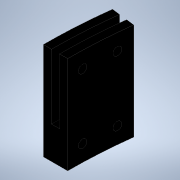
# Autodesk Inventor part: Shield Fastener
Saved by Autodesk Inventor 2020 (Build 240168000, 168)
## iProperties
Created: 2021-01-17
Part Number: Shield Fastener
Material: Generic
Document SubType Name: Modeling
Designer: magda
Density: 1 g/cm^3
Appearance: Default
Author: magda
Autodesk Inventor part; units mm, degrees
ref_plane "YZ Plane" through (0, 0, 0) normal (1, 0, 0) x (0, 1, 0)
ref_plane "XZ Plane" through (0, 0, 0) normal (0, 1, 0) x (-1, 0, 0)
ref_plane "XY Plane" through (0, 0, 0) normal (0, 0, 1) x (1, 0, 0)
sketch "Sketch1" plane through (0, 0, 0) normal (0, 1, 0) x (-1, 0, 0)
  arc A0 (207.988, -25.5377) -> (209.55, 0) centre (0, 0) ccw
  arc A1 (201.6854, -24.7639) -> (203.2, 0) centre (0, 0) ccw
  arc A2 (204.8367, -25.1508) -> (206.375, 0) centre (0, 0) ccw
  arc A3 (198.534, -24.3769) -> (200.025, 0) centre (0, 0) ccw
  line L0 (209.55, 0) -> (200.025, 0)
  line L1 (198.534, -24.3769) -> (207.988, -25.5377)
  dimension "d0" = 419.1
  dimension "d1" = 406.4
  dimension "d2" = 412.75
  dimension "d3" = 400.05
  dimension "d4" = 7
  constraints: 8 point on circle, 4 centre point, 4 coincident, 4 end point, 4 point on line, 1 horizontal
  measures "d0" diameter of A0
  measures "d1" diameter of A1
  measures "d2" diameter of A2
  measures "d3" diameter of A3
  measures "d4" angle of L1 L0
extrude "Extrusion1" add sketch "Sketch1" along normal blind 25.4 contours L1 A2 L0 A0 | L1 A3 L0 A1
ref_plane "Work Plane1" through (0, 0, 0) normal (0, -1, 0) x (1, 0, 0)
sketch "Sketch2" plane through (0, 0, 0) normal (0, -1, 0) x (1, 0, 0)
  line L0 (-203.2, 0) -> (-200.025, 0) projected
  line L1 (-209.55, 0) -> (-206.375, 0) projected
  line L2 (-200.025, 0) -> (-209.55, 0)
  line L3 (-204.8367, -25.1508) -> (-207.988, -25.5377) projected
  arc A0 (-200.025, 0) -> (-198.534, -24.3769) centre (0, 0) ccw projected
  line L4 (-207.988, -25.5377) -> (-198.534, -24.3769)
  arc A1 (-200.025, 0) -> (-198.534, -24.3769) centre (3.1749, 0.1942) ccw
  arc A2 (-209.55, 0) -> (-207.988, -25.5377) centre (0, 0) ccw projected
  arc A3 (-209.55, 0) -> (-207.988, -25.5377) centre (3.1749, 0.1942) ccw
  point P0 (-207.988, -25.5377)
  point P1 (-209.55, 0)
  constraints: 4 end point, 4 point on circle, 2 centre point, 1 collinear
extrude "Extrusion2" add sketch "Sketch2" along normal blind 12.7 contours L0 A0 L4 L3 A3 L1 L2 | A3 A2
ref_plane "Work Plane2" through (-209.55, 0, 0) normal (-0.9981348, 0, -0.0610485) x (0, 1, 0)
sketch "Sketch3" plane through (-209.55, 0, 0) normal (-0.9981348, 0, -0.0610485) x (0, 1, 0)
  circle A0 centre (19.05, 6.35) radius 1.5875
  circle A1 centre (19.05, 19.2354) radius 1.5875
  line L0 (25.4, 0) -> (-12.7, 0) projected
  line L1 (-12.7, 25.5854) -> (25.4, 25.5854) projected
  line L2 (25.4, 0) -> (25.4, 25.5854) projected
  circle A2 centre (-6.35, 19.2354) radius 1.5875
  circle A3 centre (-6.35, 6.35) radius 1.5875
  line L3 (-12.7, 25.5854) -> (-12.7, 0) projected
  point P0 (0, 12.7927)
  dimension "d10" = 3.175
  dimension "d11" = 3.175
  dimension "d12" = 6.35
  dimension "d13" = 6.35
  dimension "d14" = 6.35
  dimension "d15" = 6.35
  dimension "d16" = 3.175
  dimension "d17" = 3.175
  dimension "d18" = 6.35
  dimension "d19" = 6.35
  dimension "d20" = 6.35
  dimension "d21" = 6.35
  constraints: 4 centre point
  measures "d10" diameter of A0
  measures "d11" diameter of A1
  measures "d12" distance from line of L0 A0.centre
  measures "d13" distance from line of L1 A1.centre
  measures "d14" distance from line of A0.centre L2
  measures "d15" distance from line of A1.centre L2
  measures "d16" diameter of A2
  measures "d17" diameter of A3
  measures "d18" distance from line of L3 A3.centre
  measures "d19" distance from line of L3 A2.centre
  measures "d20" distance from line of L1 A2.centre
  measures "d21" distance from line of L0 A3.centre
extrude "Extrusion3" cut sketch "Sketch3" along normal mid plane 25.4 contours A0 | A1 | A2 | A3
body "Solid1"
